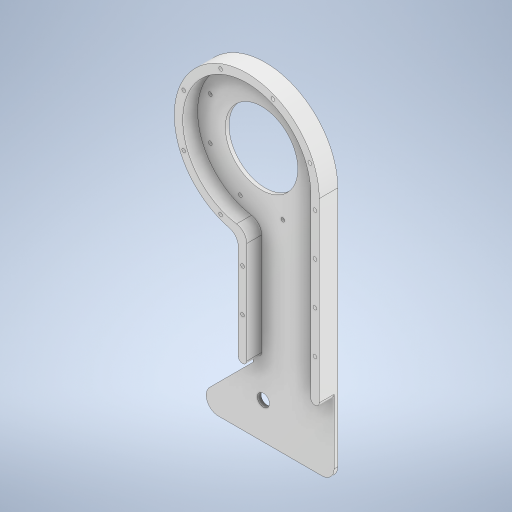
# Autodesk Inventor part: legparts_08(seven)
Saved by Autodesk Inventor 2024.3 (Build 283343000, 343)
## iProperties
Created: 2024-10-20
Part Number: legparts_08(seven)
Material: ABS プラスチック
Document SubType Name: Modeling
Designer: 佐藤智貴
Density: 1.06 g/cm^3
Appearance: 滑らか - 白
Mass: 65.0095 g
Surface Area: 440.113 cm^2
Volume: 61.3297 cm^3
Author: 佐藤智貴
Autodesk Inventor part; units mm, degrees
ref_plane "YZ Plane" through (0, 0, 0) normal (1, 0, 0) x (0, 1, 0)
ref_plane "XZ Plane" through (0, 0, 0) normal (0, 1, 0) x (-1, 0, 0)
ref_plane "XY Plane" through (0, 0, 0) normal (0, 0, 1) x (1, 0, 0)
sketch "スケッチ1" plane through (0, 0, 0) normal (0, 0, 1) x (1, 0, 0)
  circle A0 centre (0, 0) radius 60
  circle A1 centre (0, 0) radius 7
  dimension "d0" = 120
  dimension "d1" = 14
  constraints: 2 centre point, 1 coincident
  measures "d0" diameter of A0
  measures "d1" diameter of A1
extrude "押し出し1" add sketch "スケッチ1" along normal blind 3
sketch "スケッチ2" plane through (0, 0, 3) normal (0, 0, 1) x (1, 0, 0)
  circle A0 centre (0, 0) radius 46
  line L0 (0, 0) -> (0, 59.211)
  line L1 (0, 0) -> (-21.8609, 52.777)
  line L2 (0, 0) -> (27.8226, 47.8581)
  point P0 (-17.6034, 42.4985)
  point P1 (-42.4985, 17.6034)
  point P2 (-42.4985, -17.6034)
  point P3 (-17.6034, -42.4985)
  point P4 (17.6034, -42.4985)
  point P5 (42.4985, -17.6034)
  point P6 (42.4985, 17.6034)
  point P7 (17.6034, 42.4985)
  dimension "d4" = 92
  dimension "d5" = 22.5
  dimension "d8" = 360
  constraints: 6 end point, 1 coincident, 1 point on line, 1 vertical, 12 other
  measures "d5" angle of L1 L0
hole "穴1" at (-17.6034, 42.4985, 3) at (-42.4985, 17.6034, 3) at (-42.4985, -17.6034, 3) at (-17.6034, -42.4985, 3) at (17.6034, -42.4985, 3) at (42.4985, -17.6034, 3) at (42.4985, 17.6034, 3) at (17.6034, 42.4985, 3) direction (0, 0, -1) diameter 3 end through all
sketch "スケッチ4" plane through (0, 0, 0) normal (0, 0, -1) x (-1, 0, 0)
  line L0 (0, 0) -> (0, -80.557)
  circle A0 centre (0, 0) radius 60 projected
  line L1 (-60, 0) -> (-60, -210)
  line L2 (60, 0) -> (60, -210)
  line L3 (-60, -210) -> (60, -210)
  line L4 (-60, 0) -> (-41.6274, -210)
  line L5 (60, 0) -> (41.6274, -210)
  line L6 (12.7278, -162.7278) -> (60, -210)
  line L7 (19.706, -169.706) -> (-7.6224, -142.3776)
  line L8 (0, -80.557) -> (0, -150)
  line L9 (7, -239.3448) -> (7, -80.557)
  line L10 (7, -80.557) -> (7, 0)
  line L11 (7, -239.3448) -> (7, -157)
  circle A1 centre (0, 0) radius 7 projected
  point P0 (60, 0)
  point P1 (60, 0)
  point P2 (-59.0885, -10.4189)
  point P3 (-58.5, -13.3323)
  point P4 (57, -18.735)
  point P5 (59.0885, -10.4189)
  point P6 (7, -136.3384)
  point P7 (7, -59.5903)
  point P8 (43.1055, -193.1055)
  point P9 (7, -210)
  point P10 (7, -136.3384)
  point P11 (7, -157)
  dimension "d21" = 60
  dimension "d23" = 120
  dimension "d24" = 210
  dimension "d25" = 210
  dimension "d56" = 0
  dimension "d89" = 85
  dimension "d90" = 85
  dimension "d207" = 45
  dimension "d208" = 7
  constraints: 24 end point, 6 point on line, 2 vertical, 1 horizontal alignment, 1 perpendicular, 3 other
  measures "d21" distance from line of L1 L0.start
  measures "d23" distance between parallel lines of L2 L1
  measures "d24" distance of L2.start L2.end
  measures "d25" distance of L1.start L1.end
  measures "d56" angle of L2 L0
  measures "d89" angle of L3 L5
  measures "d90" angle of L3 L4
  measures "d207" angle of L3 L6
  measures "d208" distance between parallel lines of L8 L9
extrude "押し出し3" add sketch "スケッチ4" against normal blind 3 contours A0 L10 L9 L7 L8 L0 | L0 L8 L7 L9 L3 L4 A0 | L4 L3 L1 A0 | L7 L6 L5 L3 L9 | L6 L3 L5
sketch "スケッチ17" plane through (0, 0, 3) normal (0, 0, 1) x (1, 0, 0)
  circle A0 centre (0, 0) radius 30
  dimension "d159" = 60
  constraints: 1 centre point, 1 coincident
  measures "d159" diameter of A0
extrude "押し出し10" cut sketch "スケッチ17" against normal blind 10
sketch "スケッチ20" plane through (0, 0, 3) normal (0, 0, 1) x (1, 0, 0)
  line L0 (-60, -210) -> (60, -210) projected
  circle A0 centre (0, 0) radius 30 projected
  line L1 (60, -210) -> (60, 0) projected
  point P0 (1.5, -179.9937)
  point P1 (0, -210)
  point P2 (58.5, -136.6677)
  point P3 (51.5, -210)
  point P4 (48.5, -124.0626)
  point P5 (60, -150)
  dimension "d205" = 180
  dimension "d223" = 58.5
  dimension "d246" = 60
  constraints: 1 midpoint, 1 other
  measures "d205" distance of point (1.5, -179.994) A0.centre
hole "穴8" at (1.5, -179.9937, 3) direction (0, 0, -1) diameter 10 end through all
fillet "フィレット4" radius 10 2 edges at (-60, -210, 1.5) (60, -210, 1.5)
fillet "フィレット5" radius 10 2 edges at (-7, -59.5903, 1.5) (60, 0, 1.5)
sketch "スケッチ23" plane through (0, 0, 3) normal (0, 0, 1) x (1, 0, 0)
  circle A0 centre (0, 0) radius 60
  circle A1 centre (0, 0) radius 53
  arc A2 (-7, -67.9043) -> (-14.5714, -58.2037) centre (-17, -67.9043) ccw projected
  line L0 (-7, -67.9043) -> (-7, -157)
  line L1 (60, -157) -> (60, 0)
  line L2 (0, -157) -> (0, -60)
  line L3 (-7, -67.9043) -> (-7, -59.5903)
  line L4 (53, 0) -> (53, -150)
  line L5 (53, -150) -> (0, -150)
  line L6 (0, -150) -> (0, -67.9043)
  line L7 (0, -67.9043) -> (0, -59.5903)
  line L8 (53, -150) -> (53, -157)
  line L9 (0, -59.5903) -> (0, -53)
  line L10 (-35.8579, -210) -> (50, -210) projected
  line L11 (-7, -150) -> (60, -150)
  point P0 (-7, -112.4522)
  point P1 (53, 0)
  point P2 (53, -28.1247)
  dimension "d247" = 120
  dimension "d248" = 7
  dimension "d249" = 7
  dimension "d250" = 7
  dimension "d267" = 60
  constraints: 22 end point, 4 point on line, 3 point on circle, 2 tangent, 2 vertical, 1 centre point, 1 coincident, 1 midpoint, 1 parallel, 1 perpendicular, 4 other
  measures "d247" diameter of A0
  measures "d249" distance from line of point (-7, -112.452) L2
  measures "d250" distance between parallel lines of L0 L6
  measures "d267" distance between parallel lines of L10 L5
extrude "押し出し14" add sketch "スケッチ23" along normal blind 12.3 contours A0 L4 A1 L9 L7 | L1 L11 L4 A0 | A0 L3 A2 | A0 L2 L11 L0 L3 picked at (54.2848, -15.7658)
sketch "スケッチ24" plane through (0, 0, 15.3) normal (0, 0, 1) x (1, 0, 0)
  circle A0 centre (0, 0) radius 60
  circle A1 centre (0, 0) radius 56.5
  circle A2 centre (-17.6034, 42.4985) radius 1.5 projected
  line L0 (0, 0) -> (-17.6034, 42.4985)
  line L1 (-17.6034, 42.4985) -> (-25.261, 60.9855)
  point P0 (-21.6216, 52.1992)
  point P1 (-52.1992, 21.6216)
  point P2 (-52.1992, -21.6216)
  point P3 (-21.6216, -52.1992)
  point P4 (21.6216, -52.1992)
  point P5 (52.1992, -21.6216)
  point P6 (52.1992, 21.6216)
  point P7 (21.6216, 52.1992)
  dimension "d253" = 120
  dimension "d254" = 3.5
  dimension "d257" = 360
  constraints: 4 end point, 2 point on line, 1 centre point, 1 coincident, 12 other
  measures "d253" diameter of A0
hole "穴10" at (-21.6216, -52.1992, 15.3) at (-52.1992, -21.6216, 15.3) at (-52.1992, 21.6216, 15.3) at (-21.6216, 52.1992, 15.3) at (21.6216, 52.1992, 15.3) at (52.1992, 21.6216, 15.3) direction (0, 0, -1) diameter 3 end through all
sketch "スケッチ25" plane through (0, 0, 15.3) normal (0, 0, 1) x (1, 0, 0)
  line L0 (-7, -150) -> (0, -150) projected
  line L1 (-7, -67.9043) -> (-7, -150) projected
  line L2 (60, -150) -> (60, 0) projected
  line L3 (53, -150) -> (60, -150) projected
  point P0 (0, 0)
  point P1 (-3.5, -80)
  point P2 (56.5, -80)
  point P3 (-3.5, -115)
  point P4 (56.5, -115)
  point P5 (56.5, -45)
  point P6 (56.5, -10)
  point P7 (-3.5, -150)
  point P8 (56.5, -150)
  dimension "d268" = 35
  dimension "d269" = 35
  dimension "d270" = 3.5
  dimension "d271" = 3.5
  dimension "d272" = 3.5
  dimension "d273" = 3.5
  dimension "d274" = 3.5
  dimension "d275" = 3.5
  dimension "d276" = 35
  dimension "d277" = 35
  dimension "d278" = 35
  dimension "d279" = 35
  constraints: 2 midpoint
  measures "d268" distance of point (-3.5, -80) point (-3.5, -115)
  measures "d269" distance of point (-3.5, -150) point (-3.5, -115)
  measures "d270" distance from line of L1 point (-3.5, -115)
  measures "d271" distance from line of L1 point (-3.5, -80)
  measures "d272" distance from line of L2 point (56.5, -115)
  measures "d273" distance from line of L2 point (56.5, -80)
  measures "d274" distance from line of L2 point (56.5, -45)
  measures "d275" distance from line of L2 point (56.5, -10)
  measures "d276" distance of point (56.5, -150) point (56.5, -115)
  measures "d277" distance of point (56.5, -115) point (56.5, -80)
  measures "d278" distance of point (56.5, -80) point (56.5, -45)
  measures "d279" distance of point (56.5, -45) point (56.5, -10)
hole "穴11" at (-3.5, -80, 15.3) at (56.5, -80, 15.3) at (-3.5, -115, 15.3) at (56.5, -115, 15.3) at (56.5, -45, 15.3) at (56.5, -10, 15.3) direction (0, 0, -1) diameter 3 end through all
fillet "フィレット8" radius 3.5 4 edges at (-7, -150, 9.15) (0, -150, 9.15) (53, -150, 9.15) (60, -150, 9.15)
fillet "フィレット9" radius 10 1 edges at (0, -53, 9.15)
equation "\"d25\" = d24"
equation "\"d90\" = d89"
